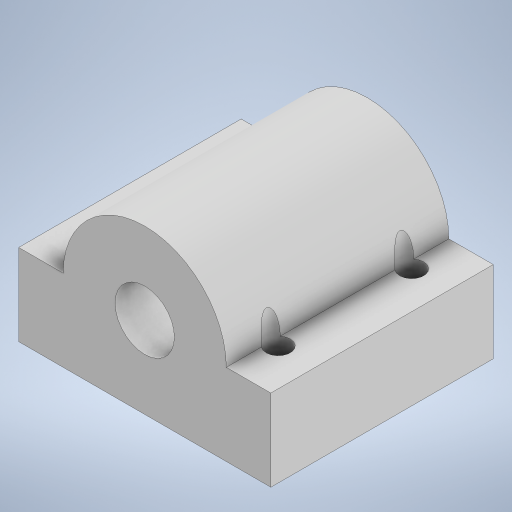
# Autodesk Inventor part: Pillow block bearing
Saved by Autodesk Inventor 2023.1 (Build 271208000, 208)
## iProperties
Created: 2022-10-30
Part Number: Pillow block bearing
Material: Generic
Document SubType Name: Modeling
Designer: nicol
Density: 1 g/cm^3
Appearance: Default
Author: nicol
Autodesk Inventor part; units mm, degrees
ref_plane "YZ Plane" through (0, 0, 0) normal (1, 0, 0) x (0, 1, 0)
ref_plane "XZ Plane" through (0, 0, 0) normal (0, 1, 0) x (-1, 0, 0)
ref_plane "XY Plane" through (0, 0, 0) normal (0, 0, 1) x (1, 0, 0)
sketch "Sketch1" plane through (0, 0, 0) normal (0, 0, 1) x (1, 0, 0)
  line L0 (0, 0) -> (34, 0)
  line L1 (34, 0) -> (34, 11)
  line L2 (34, 11) -> (0, 11)
  line L3 (0, 11) -> (0, 0)
  circle A0 centre (17, 11) radius 11
  circle A1 centre (17, 11) radius 4
  line L4 (9.5554, 22) -> (24.3175, 22)
  point P0 (28, 11)
  point P1 (6, 11)
  dimension "d0" = 34
  dimension "d1" = 11
  dimension "d3" = 8
  dimension "d4" = 22
  constraints: 10 end point, 2 centre point, 2 coincident, 2 horizontal, 2 parallel, 1 midpoint, 1 perpendicular, 1 tangent
  measures "d0" distance of L0.start L0.end
  measures "d1" distance between parallel lines of L0 L2
  measures "d3" diameter of A1
  measures "d4" distance between parallel lines of L0 L4
extrude "Extrusion1" add sketch "Sketch1" along normal blind 30 contours L3 L2 A0 L0 | A0 L2 L1 L0 | A0 L2 A1 | A0 L2 A1
sketch "Sketch2" plane through (0, 0, 0) normal (0, -1, 0) x (1, 0, 0)
  line L0 (34, 0) -> (34, 30) projected
  line L1 (0, 0) -> (0, 30) projected
  line L2 (0, 0) -> (34, 0) projected
  line L3 (0, 30) -> (34, 30) projected
  point P0 (5, 24)
  point P1 (29, 24)
  point P2 (29, 6)
  point P3 (5, 6)
  dimension "d7" = 24
  dimension "d8" = 18
  dimension "d9" = 5
  dimension "d10" = 5
  dimension "d11" = 6
  dimension "d12" = 6
  constraints: 2 horizontal alignment, 2 vertical alignment
  measures "d7" distance of point (29, 24) point (5, 24)
  measures "d8" distance of point (29, 6) point (29, 24)
  measures "d9" distance from line of L0 point (29, 24)
  measures "d10" distance from line of L1 point (5, 24)
  measures "d11" distance from line of L2 point (29, 6)
  measures "d12" distance from line of L3 point (29, 24)
hole "Hole1" at (5, 0, 24) at (29, 0, 24) at (29, 0, 6) at (5, 0, 6) direction (0, 1, 0) diameter 3.242 end through all thread size "M4x0.7" class "6H" standard "ANSI Metric M Profile"
equation "\"d9\" = d10"
equation "\"d11\" = d12"
body "Solid1"
